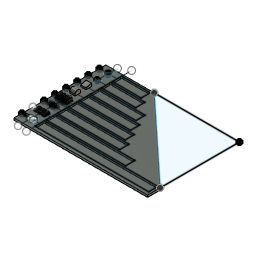
tactileMapsLegend (Autodesk Fusion 360 archive; units mm, degrees)
design "tactileMapsLegendApril26" references "TactileMapsParameters"
Autodesk Fusion 360 part; units mm, degrees
derive "ExternalDerived1" from "TactileMapsParameters v7"
sketch "Sketch1" plane through (0, 0, 0) normal (0, 0, 1) x (1, 0, 0)
  line L0 (0, 0) -> (147.25, 0)
  line L1 (147.25, 0) -> (147.25, 101.2)
  line L2 (147.25, 101.2) -> (0, 101.2)
  line L3 (0, 101.2) -> (0, 0)
  dimension "d21" = 147.25
  dimension "d22" = 101.2
  constraint horizontal L0
  constraint vertical L1
  constraint horizontal L2
  constraint vertical L3
  constraint coincident L0.start L3.end
  measures "d21" distance of L0.start L0.end
  measures "d22" distance of L0.start L2.end
extrude "Extrude1" add sketch "Sketch1" along normal blind 2.2
sketch "Sketch2" plane through (0, 0, 2.2) normal (0, 0, 1) x (-1, 0, 0)
  line L0 (0, -101.2) -> (0, 0)
  line L1 (0, 0) -> (-147.25, 0)
  line L2 (-147.25, 0) -> (-147.25, -101.2)
  line L3 (-147.25, -101.2) -> (0, -101.2)
  line L4 (-19.6, -110.066) -> (-19.6, 6.0036) construction
  line L5 (-19.6, -99.2) -> (-51.05, -99.2)
  line L6 (-51.05, -99.2) -> (-51.05, -89)
  line L7 (-51.05, -89) -> (-19.6, -89)
  line L8 (-19.6, -89) -> (-19.6, -99.2)
  line L9 (-19.6, -87) -> (-57.3, -87)
  line L10 (-57.3, -87) -> (-57.3, -76.8)
  line L11 (-57.3, -76.8) -> (-19.6, -76.8)
  line L12 (-19.6, -76.8) -> (-19.6, -87)
  line L13 (-19.6, -74.8) -> (-69.8, -74.8)
  line L14 (-69.8, -74.8) -> (-69.8, -64.6)
  line L15 (-69.8, -64.6) -> (-19.6, -64.6)
  line L16 (-19.6, -64.6) -> (-19.6, -74.8)
  line L17 (-19.6, -62.6) -> (-76.05, -62.6)
  line L18 (-76.05, -62.6) -> (-76.05, -52.4)
  line L19 (-76.05, -52.4) -> (-19.6, -52.4)
  line L20 (-19.6, -52.4) -> (-19.6, -62.6)
  line L21 (-19.6, -50.4) -> (-82.3, -50.4)
  line L22 (-82.3, -50.4) -> (-82.3, -40.2)
  line L23 (-82.3, -40.2) -> (-19.6, -40.2)
  line L24 (-19.6, -40.2) -> (-19.6, -50.4)
  line L25 (-19.6, -38.2) -> (-88.55, -38.2)
  line L26 (-88.55, -38.2) -> (-88.55, -28)
  line L27 (-88.55, -28) -> (-19.6, -28)
  line L28 (-19.6, -28) -> (-19.6, -38.2)
  line L29 (-19.6, -26) -> (-107.3, -26)
  line L30 (-107.3, -26) -> (-107.3, -15.8)
  line L31 (-107.3, -15.8) -> (-19.6, -15.8)
  line L32 (-19.6, -15.8) -> (-19.6, -26)
  line L33 (-19.6, -13.8) -> (-144.8, -13.8)
  line L34 (-144.8, -13.8) -> (-144.8, -3.6)
  line L35 (-144.8, -3.6) -> (-19.6, -3.6)
  line L36 (-19.6, -3.6) -> (-19.6, -13.8)
  line L37 (-19.6, -94.1) -> (0, -94.1) construction
  line L38 (-19.6, -81.9) -> (0, -81.9) construction
  line L39 (-19.6, -69.7) -> (0, -69.7) construction
  line L40 (-19.6, -57.5) -> (0, -57.5) construction
  line L41 (-19.6, -45.3) -> (0, -45.3) construction
  line L42 (-19.6, -33.1) -> (0, -33.1) construction
  line L43 (-19.6, -20.9) -> (0, -20.9) construction
  line L44 (-19.6, -8.7) -> (0, -8.7) construction
  line L45 (-11.8835, -96.2585) -> (-9.747, -97.0995)
  line L46 (-9.747, -97.0995) -> (-7.6415, -96.1835)
  line L47 (-7.6415, -96.1835) -> (-6.8005, -94.047)
  line L48 (-6.8005, -94.047) -> (-7.7165, -91.9415)
  line L49 (-7.7165, -91.9415) -> (-9.853, -91.1005)
  line L50 (-9.853, -91.1005) -> (-11.9585, -92.0165)
  line L51 (-11.9585, -92.0165) -> (-12.7995, -94.153)
  line L52 (-12.7995, -94.153) -> (-11.8835, -96.2585)
  line L53 (-12.3958, -83.4039) -> (-7.1997, -83.3961)
  line L54 (-7.1997, -83.3961) -> (-9.8045, -78.9)
  line L55 (-9.8045, -78.9) -> (-12.3958, -83.4039)
  line L56 (-15.8, -48.3) -> (-3.8, -48.3)
  line L57 (-3.8, -48.3) -> (-3.8, -42.3)
  line L58 (-3.8, -42.3) -> (-15.8, -42.3)
  line L59 (-15.8, -42.3) -> (-15.8, -48.3)
  line L60 (-15.8, -48.3) -> (-3.8, -42.3) construction
  line L61 (-3.8, -48.3) -> (-15.8, -42.3) construction
  line L62 (-3.8, -48.3) -> (-5.3, -48.3)
  line L63 (-5.3, -48.3) -> (-5.3, -42.3)
  line L64 (-5.3, -42.3) -> (-3.8, -42.3)
  line L65 (-3.8, -42.3) -> (-3.8, -48.3)
  line L66 (-8.8, -48.3) -> (-8.8, -42.3)
  line L67 (-7.3, -48.3) -> (-7.3, -42.3)
  line L68 (-7.3, -48.3) -> (-8.8, -48.3)
  line L69 (-8.8, -42.3) -> (-7.3, -42.3)
  line L70 (-12.3, -48.3) -> (-12.3, -42.3)
  line L71 (-10.8, -48.3) -> (-10.8, -42.3)
  line L72 (-10.8, -48.3) -> (-12.3, -48.3)
  line L73 (-12.3, -42.3) -> (-10.8, -42.3)
  line L74 (-15.8, -48.3) -> (-15.8, -42.3)
  line L75 (-14.3, -48.3) -> (-14.3, -42.3)
  line L76 (-14.3, -48.3) -> (-15.8, -48.3)
  line L77 (-15.8, -42.3) -> (-14.3, -42.3)
  circle A0 centre (-9.8, -33.1) radius 0.75
  circle A1 centre (-12.8, -33.1) radius 0.75
  circle A2 centre (-6.8, -33.1) radius 0.75
  line L78 (-3.8, -23.4) -> (-15.8, -23.4)
  line L79 (-15.8, -23.4) -> (-15.8, -21.9)
  line L80 (-15.8, -21.9) -> (-3.8, -21.9)
  line L81 (-3.8, -21.9) -> (-3.8, -23.4)
  line L82 (-15.8, -19.9) -> (-3.8, -19.9)
  line L83 (-3.8, -19.9) -> (-3.8, -18.4)
  line L84 (-3.8, -18.4) -> (-15.8, -18.4)
  line L85 (-15.8, -18.4) -> (-15.8, -19.9)
  line L86 (-4.8, -23.9) -> (-6.3, -23.9)
  line L87 (-6.3, -23.9) -> (-6.3, -17.9)
  line L88 (-6.3, -17.9) -> (-4.8, -17.9)
  line L89 (-4.8, -17.9) -> (-4.8, -23.9)
  line L90 (-10.55, -23.9) -> (-10.55, -17.9)
  line L91 (-9.05, -23.9) -> (-10.55, -23.9)
  line L92 (-9.05, -17.9) -> (-9.05, -23.9)
  line L93 (-10.55, -17.9) -> (-9.05, -17.9)
  line L94 (-14.8, -23.9) -> (-14.8, -17.9)
  line L95 (-13.3, -23.9) -> (-14.8, -23.9)
  line L96 (-13.3, -17.9) -> (-13.3, -23.9)
  line L97 (-14.8, -17.9) -> (-13.3, -17.9)
  line L98 (-3.8, -9.7) -> (-9.9716, -9.7)
  line L99 (-9.9716, -7.7) -> (-3.8, -7.7)
  line L100 (-3.8, -7.7) -> (-3.8, -9.7)
  arc A3 (-9.9716, -7.7) -> (-9.9716, -9.7) centre (-12.8, -8.7) ccw
  line L101 (-9.8, -104.251) -> (-9.8, -8.7) construction
  line L102 (-9.8, -7.7) -> (-9.8, 5.278) construction
  line L103 (-53.2749, -101.2) -> (-147.25, -13.8)
  line L104 (-147.25, -13.8) -> (-147.25, -101.2)
  line L105 (-147.25, -101.2) -> (-53.2749, -101.2)
  point P0 (-9.8, -94.1)
  point P1 (-9.8, -81.9)
  point P2 (-9.8, -45.3)
  dimension "d25" = 19.6
  dimension "d26" = 31.45
  dimension "d27" = 10.2
  dimension "d28" = 2
  dimension "d29" = 37.7
  dimension "d30" = 2
  dimension "d31" = 10.2
  dimension "d32" = 50.2
  dimension "d33" = 10.2
  dimension "d34" = 2
  dimension "d35" = 56.45
  dimension "d36" = 10.2
  dimension "d37" = 2
  dimension "d38" = 62.7
  dimension "d39" = 10.2
  dimension "d40" = 2
  dimension "d41" = 68.95
  dimension "d42" = 10.2
  dimension "d43" = 2
  dimension "d44" = 87.7
  dimension "d45" = 10.2
  dimension "d46" = 2
  dimension "d47" = 125.2
  dimension "d48" = 10.2
  dimension "d49" = 2
  dimension "d50" = 9.8
  dimension "d51" = 3
  dimension "d52" = 3
  dimension "d53" = 12
  dimension "d54" = 6
  dimension "d55" = 1.5
  dimension "d56" = 6
  dimension "d59" = -10.5
  dimension "d60" = 0
  dimension "d61" = 1.5
  dimension "d64" = 3
  dimension "d65" = 0
  dimension "d66" = 12
  dimension "d67" = 1.5
  dimension "d68" = 6
  dimension "d69" = 2.5
  dimension "d70" = 1.5
  dimension "d71" = 6
  dimension "d72" = 0.5
  dimension "d73" = 1
  dimension "d76" = -8.5
  dimension "d77" = 0
  dimension "d78" = 6
  dimension "d83" = 2
  dimension "d84" = 1
  dimension "d85" = 6
  constraint perpendicular L1 L4
  constraint horizontal L5
  constraint vertical L6
  constraint horizontal L7
  constraint vertical L8
  constraint coincident L4 L5.start
  constraint horizontal L9
  constraint vertical L10
  constraint horizontal L11
  constraint vertical L12
  constraint coincident L4 L9.start
  constraint horizontal L13
  constraint vertical L14
  constraint horizontal L15
  constraint vertical L16
  constraint coincident L4 L13.start
  constraint horizontal L17
  constraint vertical L18
  constraint horizontal L19
  constraint vertical L20
  constraint coincident L4 L17.start
  constraint horizontal L21
  constraint vertical L22
  constraint horizontal L23
  constraint vertical L24
  constraint coincident L4 L21.start
  constraint horizontal L25
  constraint vertical L26
  constraint horizontal L27
  constraint vertical L28
  constraint coincident L4 L25.start
  constraint horizontal L29
  constraint vertical L30
  constraint horizontal L31
  constraint vertical L32
  constraint coincident L4 L29.start
  constraint horizontal L33
  constraint vertical L34
  constraint horizontal L35
  constraint vertical L36
  constraint coincident L4 L33.start
  constraint perpendicular L1 L101
  constraint midpoint L8 L37.start
  constraint coincident L0 L37.end
  constraint perpendicular L0 L37
  constraint midpoint L12 L38.start
  constraint coincident L0 L38.end
  constraint perpendicular L0 L38
  constraint midpoint L16 L39.start
  constraint coincident L0 L39.end
  constraint perpendicular L0 L39
  constraint midpoint L20 L40.start
  constraint coincident L0 L40.end
  constraint perpendicular L0 L40
  constraint midpoint L24 L41.start
  constraint coincident L0 L41.end
  constraint perpendicular L0 L41
  constraint midpoint L28 L42.start
  constraint coincident L0 L42.end
  constraint perpendicular L0 L42
  constraint midpoint L32 L43.start
  constraint perpendicular L32 L43
  constraint midpoint L36 L44.start
  constraint coincident L0 L44.end
  constraint perpendicular L0 L44
  constraint midpoint L37 P0
  constraint midpoint L38 P1
  constraint horizontal L56
  constraint perpendicular L56 L57
  constraint parallel L56 L58
  constraint parallel L57 L59
  constraint coincident L60 P2
  constraint coincident L61 P2
  constraint midpoint L41 P2
  constraint horizontal L62
  constraint vertical L63
  constraint horizontal L64
  constraint vertical L65
  constraint midpoint L42 A0.centre
  constraint horizontal L78
  constraint vertical L79
  constraint horizontal L80
  constraint vertical L81
  constraint symmetric L43 L78.start L83.end
  constraint symmetric L43 L78.end L84.end
  constraint symmetric L43 L79.end L82.start
  constraint symmetric L43 L80.end L82.end
  constraint horizontal L86
  constraint vertical L87
  constraint horizontal L88
  constraint vertical L89
  constraint horizontal L98
  constraint horizontal L99
  constraint vertical L100
  constraint coincident L102.start L99
  constraint collinear L101 L102
  constraint coincident L3 L103.start
  constraint coincident L2 L103.end
  constraint coincident L2.end L3.start
  measures "d25" distance of L0 L4
  measures "d26" distance of L5.start L5.end
  measures "d27" distance of L5.start L7.end
  measures "d28" distance of L3 L5
  measures "d29" distance of L9.start L9.end
  measures "d30" distance of L7 L9
  measures "d31" distance of L9.end L10.end
  measures "d32" distance of L13.start L13.end
  measures "d33" distance of L13.start L15.end
  measures "d34" distance of L11 L13
  measures "d35" distance of L17.start L17.end
  measures "d36" distance of L17.start L19.end
  measures "d37" distance of L15 L17
  measures "d38" distance of L21.start L21.end
  measures "d39" distance of L21.start L23.end
  measures "d40" distance of L19 L21
  measures "d41" distance of L25.start L25.end
  measures "d42" distance of L25.start L27.end
  measures "d43" distance of L23 L25
  measures "d44" distance of L29.start L29.end
  measures "d45" distance of L29.start L31.end
  measures "d46" distance of L27 L29
  measures "d47" distance of L33.start L33.end
  measures "d48" distance of L33.start L35.end
  measures "d49" distance of L31 L33
  measures "d50" distance of L0.start L101
  measures "d51" distance of L45.start P0
  measures "d52" distance of L53.start P1
  measures "d53" distance of L57.end L58.end
  measures "d54" distance of L56.end L57.end
  measures "d55" distance of L56.end L62.end
  measures "d56" distance of L56.end L57.end
  measures "d61" diameter of A0
  measures "d66" distance of L78.start L78.end
  measures "d67" distance of L78.start L80.end
  measures "d68" distance of L81 L101
  measures "d69" distance of L43 L78
  measures "d70" distance of L86.start L86.end
  measures "d71" distance of L86.start L88.end
  measures "d72" distance of L78 L86
  measures "d73" distance of L83 L89
  measures "d78" diameter of A3
  measures "d83" distance of L98.start L99.end
  measures "d84" distance of L44 L98
  measures "d85" distance of L100 L101
extrude "Extrude2" cut sketch "Sketch2" against normal blind 2 contours L5 L6 L7 L8 | L9 L10 L11 L12 | L13 L14 L15 L16 | L17 L18 L19 L20 | L21 L22 L23 L24 | L25 L26 L27 L28 | L29 L30 L31 L32 | L33 L34 L35 L36
ref_plane "WorkPlane1" through (88.55, 38.2, 2.2) normal (0, 0, -1) x (-1, 0, 0)
sketch "Sketch3" plane through (88.55, 38.2, 2.2) normal (0, 0, -1) x (-1, 0, 0)
  line L0 (68.95, 0) -> (0, 0) construction
  line L1 (0, 0) -> (0, -10.2) construction
  line L2 (0, 0) -> (0.7071, -0.7071) construction
  circle A0 centre (0.7071, -0.7071) radius 1
  dimension "d89" = 1
  constraint coincident L0.end L1.start
  constraint coincident L0.end A0
  measures "d89" distance of L0.end L2.end
sweep "Sweep1" cut kept parallel profiles "Sketch3" along 1 edges at (88.55, 38.2, 1.2) section 1
ref_plane "WorkPlane2" through (88.55, 28, 2.2) normal (0, 0, -1) x (-1, 0, 0)
sketch "Sketch4" plane through (88.55, 28, 2.2) normal (0, 0, -1) x (-1, 0, 0)
  line L0 (0, 0) -> (68.95, 0) construction
  line L1 (0, 8.7858) -> (0, 0) construction
  line L2 (0, 0) -> (0.7071, 0.7071) construction
  circle A0 centre (0.7071, 0.7071) radius 1
  dimension "d97" = 1
  constraint coincident L0.start L1.end
  constraint coincident L0.start A0
  measures "d97" distance of L0.start L2.end
sweep "Sweep2" cut kept parallel profiles "Sketch4" along 1 edges at (88.55, 28, 1.2) section 1
ref_plane "WorkPlane3" through (19.6, 38.2, 2.2) normal (0, 0, -1) x (-1, 0, 0)
sketch "Sketch5" plane through (19.6, 38.2, 2.2) normal (0, 0, -1) x (-1, 0, 0)
  line L0 (0, -10.2) -> (0, 0) construction
  line L1 (0, 0) -> (-67.5358, 0) construction
  line L2 (0, 0) -> (-0.7071, -0.7071) construction
  circle A0 centre (-0.7071, -0.7071) radius 1
  dimension "d105" = 1
  constraint coincident L0.end L1.start
  constraint coincident L0.end A0
  measures "d105" distance of L0.end L2.end
sweep "Sweep3" cut kept parallel profiles "Sketch5" along 1 edges at (19.6, 38.2, 1.2) section 1
ref_plane "WorkPlane4" through (19.6, 28, 2.2) normal (0, 0, -1) x (-1, 0, 0)
sketch "Sketch6" plane through (19.6, 28, 2.2) normal (0, 0, -1) x (-1, 0, 0)
  line L0 (-67.5358, 0) -> (0, 0) construction
  line L1 (0, 0) -> (0, 8.7858) construction
  line L2 (0, 0) -> (-0.7071, 0.7071) construction
  circle A0 centre (-0.7071, 0.7071) radius 1
  dimension "d113" = 1
  constraint coincident L0.end L1.start
  constraint coincident L0.end A0
  measures "d113" distance of L0.end L2.end
sweep "Sweep4" cut kept parallel profiles "Sketch6" along 1 edges at (19.6, 28, 1.2) section 1
ref_plane "WorkPlane5" through (57.3, 87, 2.2) normal (0, 0, -1) x (-1, 0, 0)
sketch "Sketch7" plane through (57.3, 87, 2.2) normal (0, 0, -1) x (-1, 0, 0)
  line L0 (37.7, 0) -> (0, 0) construction
  line L1 (0, 0) -> (0, -10.2) construction
  line L2 (0, 0) -> (0.7071, -0.7071) construction
  circle A0 centre (0.7071, -0.7071) radius 1
  dimension "d121" = 1
  constraint coincident L0.end L1.start
  constraint coincident L0.end A0
  measures "d121" distance of L0.end L2.end
sweep "Sweep5" cut kept parallel profiles "Sketch7" along 1 edges at (57.3, 87, 1.2) section 1
ref_plane "WorkPlane6" through (57.3, 76.8, 2.2) normal (0, 0, -1) x (-1, 0, 0)
sketch "Sketch8" plane through (57.3, 76.8, 2.2) normal (0, 0, -1) x (-1, 0, 0)
  line L0 (0, 0) -> (37.7, 0) construction
  line L1 (0, 8.7858) -> (0, 0) construction
  line L2 (0, 0) -> (0.7071, 0.7071) construction
  circle A0 centre (0.7071, 0.7071) radius 1
  dimension "d129" = 1
  constraint coincident L0.start L1.end
  constraint coincident L0.start A0
  measures "d129" distance of L0.start L2.end
sweep "Sweep6" cut kept parallel profiles "Sketch8" along 1 edges at (57.3, 76.8, 1.2) section 1
ref_plane "WorkPlane7" through (19.6, 87, 2.2) normal (0, 0, -1) x (-1, 0, 0)
sketch "Sketch9" plane through (19.6, 87, 2.2) normal (0, 0, -1) x (-1, 0, 0)
  line L0 (0, -10.2) -> (0, 0) construction
  line L1 (0, 0) -> (-36.2858, 0) construction
  line L2 (0, 0) -> (-0.7071, -0.7071) construction
  circle A0 centre (-0.7071, -0.7071) radius 1
  dimension "d137" = 1
  constraint coincident L0.end L1.start
  constraint coincident L0.end A0
  measures "d137" distance of L0.end L2.end
sweep "Sweep7" cut kept parallel profiles "Sketch9" along 1 edges at (19.6, 87, 1.2) section 1
ref_plane "WorkPlane8" through (19.6, 76.8, 2.2) normal (0, 0, -1) x (-1, 0, 0)
sketch "Sketch10" plane through (19.6, 76.8, 2.2) normal (0, 0, -1) x (-1, 0, 0)
  line L0 (-36.2858, 0) -> (0, 0) construction
  line L1 (0, 0) -> (0, 8.7858) construction
  line L2 (0, 0) -> (-0.7071, 0.7071) construction
  circle A0 centre (-0.7071, 0.7071) radius 1
  dimension "d145" = 1
  constraint coincident L0.end L1.start
  constraint coincident L0.end A0
  measures "d145" distance of L0.end L2.end
sweep "Sweep8" cut kept parallel profiles "Sketch10" along 1 edges at (19.6, 76.8, 1.2) section 1
ref_plane "WorkPlane9" through (69.8, 74.8, 2.2) normal (0, 0, -1) x (-1, 0, 0)
sketch "Sketch11" plane through (69.8, 74.8, 2.2) normal (0, 0, -1) x (-1, 0, 0)
  line L0 (50.2, 0) -> (0, 0) construction
  line L1 (0, 0) -> (0, -10.2) construction
  line L2 (0, 0) -> (0.7071, -0.7071) construction
  circle A0 centre (0.7071, -0.7071) radius 1
  dimension "d153" = 1
  constraint coincident L0.end L1.start
  constraint coincident L0.end A0
  measures "d153" distance of L0.end L2.end
sweep "Sweep9" cut kept parallel profiles "Sketch11" along 1 edges at (69.8, 74.8, 1.2) section 1
ref_plane "WorkPlane10" through (69.8, 64.6, 2.2) normal (0, 0, -1) x (-1, 0, 0)
sketch "Sketch12" plane through (69.8, 64.6, 2.2) normal (0, 0, -1) x (-1, 0, 0)
  line L0 (0, 0) -> (50.2, 0) construction
  line L1 (0, 8.7858) -> (0, 0) construction
  line L2 (0, 0) -> (0.7071, 0.7071) construction
  circle A0 centre (0.7071, 0.7071) radius 1
  dimension "d161" = 1
  constraint coincident L0.start L1.end
  constraint coincident L0.start A0
  measures "d161" distance of L0.start L2.end
sweep "Sweep10" cut kept parallel profiles "Sketch12" along 1 edges at (69.8, 64.6, 1.2) section 1
ref_plane "WorkPlane11" through (19.6, 74.8, 2.2) normal (0, 0, -1) x (-1, 0, 0)
sketch "Sketch13" plane through (19.6, 74.8, 2.2) normal (0, 0, -1) x (-1, 0, 0)
  line L0 (0, -10.2) -> (0, 0) construction
  line L1 (0, 0) -> (-48.7858, 0) construction
  line L2 (0, 0) -> (-0.7071, -0.7071) construction
  circle A0 centre (-0.7071, -0.7071) radius 1
  dimension "d169" = 1
  constraint coincident L0.end L1.start
  constraint coincident L0.end A0
  measures "d169" distance of L0.end L2.end
sweep "Sweep11" cut kept parallel profiles "Sketch13" along 1 edges at (19.6, 74.8, 1.2) section 1
ref_plane "WorkPlane12" through (19.6, 64.6, 2.2) normal (0, 0, -1) x (-1, 0, 0)
sketch "Sketch14" plane through (19.6, 64.6, 2.2) normal (0, 0, -1) x (-1, 0, 0)
  line L0 (-48.7858, 0) -> (0, 0) construction
  line L1 (0, 0) -> (0, 8.7858) construction
  line L2 (0, 0) -> (-0.7071, 0.7071) construction
  circle A0 centre (-0.7071, 0.7071) radius 1
  dimension "d177" = 1
  constraint coincident L0.end L1.start
  constraint coincident L0.end A0
  measures "d177" distance of L0.end L2.end
sweep "Sweep12" cut kept parallel profiles "Sketch14" along 1 edges at (19.6, 64.6, 1.2) section 1
ref_plane "WorkPlane13" through (107.3, 26, 2.2) normal (0, 0, -1) x (-1, 0, 0)
sketch "Sketch15" plane through (107.3, 26, 2.2) normal (0, 0, -1) x (-1, 0, 0)
  line L0 (87.7, 0) -> (0, 0) construction
  line L1 (0, 0) -> (0, -10.2) construction
  line L2 (0, 0) -> (0.7071, -0.7071) construction
  circle A0 centre (0.7071, -0.7071) radius 1
  dimension "d185" = 1
  constraint coincident L0.end L1.start
  constraint coincident L0.end A0
  measures "d185" distance of L0.end L2.end
sweep "Sweep13" cut kept parallel profiles "Sketch15" along 1 edges at (107.3, 26, 1.2) section 1
ref_plane "WorkPlane14" through (107.3, 15.8, 2.2) normal (0, 0, -1) x (-1, 0, 0)
sketch "Sketch16" plane through (107.3, 15.8, 2.2) normal (0, 0, -1) x (-1, 0, 0)
  line L0 (0, 0) -> (87.7, 0) construction
  line L1 (0, 8.7858) -> (0, 0) construction
  line L2 (0, 0) -> (0.7071, 0.7071) construction
  circle A0 centre (0.7071, 0.7071) radius 1
  dimension "d193" = 1
  constraint coincident L0.start L1.end
  constraint coincident L0.start A0
  measures "d193" distance of L0.start L2.end
sweep "Sweep14" cut kept parallel profiles "Sketch16" along 1 edges at (107.3, 15.8, 1.2) section 1
ref_plane "WorkPlane15" through (19.6, 26, 2.2) normal (0, 0, -1) x (-1, 0, 0)
sketch "Sketch17" plane through (19.6, 26, 2.2) normal (0, 0, -1) x (-1, 0, 0)
  line L0 (0, -10.2) -> (0, 0) construction
  line L1 (0, 0) -> (-86.2858, 0) construction
  line L2 (0, 0) -> (-0.7071, -0.7071) construction
  circle A0 centre (-0.7071, -0.7071) radius 1
  dimension "d201" = 1
  constraint coincident L0.end L1.start
  constraint coincident L0.end A0
  measures "d201" distance of L0.end L2.end
sweep "Sweep15" cut kept parallel profiles "Sketch17" along 1 edges at (19.6, 26, 1.2) section 1
ref_plane "WorkPlane16" through (19.6, 15.8, 2.2) normal (0, 0, -1) x (-1, 0, 0)
sketch "Sketch18" plane through (19.6, 15.8, 2.2) normal (0, 0, -1) x (-1, 0, 0)
  line L0 (-86.2858, 0) -> (0, 0) construction
  line L1 (0, 0) -> (0, 8.7858) construction
  line L2 (0, 0) -> (-0.7071, 0.7071) construction
  circle A0 centre (-0.7071, 0.7071) radius 1
  dimension "d209" = 1
  constraint coincident L0.end L1.start
  constraint coincident L0.end A0
  measures "d209" distance of L0.end L2.end
sweep "Sweep16" cut kept parallel profiles "Sketch18" along 1 edges at (19.6, 15.8, 1.2) section 1
ref_plane "WorkPlane17" through (82.3, 50.4, 2.2) normal (0, 0, -1) x (-1, 0, 0)
sketch "Sketch19" plane through (82.3, 50.4, 2.2) normal (0, 0, -1) x (-1, 0, 0)
  line L0 (62.7, 0) -> (0, 0) construction
  line L1 (0, 0) -> (0, -10.2) construction
  line L2 (0, 0) -> (0.7071, -0.7071) construction
  circle A0 centre (0.7071, -0.7071) radius 1
  dimension "d217" = 1
  constraint coincident L0.end L1.start
  constraint coincident L0.end A0
  measures "d217" distance of L0.end L2.end
sweep "Sweep17" cut kept parallel profiles "Sketch19" along 1 edges at (82.3, 50.4, 1.2) section 1
ref_plane "WorkPlane18" through (82.3, 40.2, 2.2) normal (0, 0, -1) x (-1, 0, 0)
sketch "Sketch20" plane through (82.3, 40.2, 2.2) normal (0, 0, -1) x (-1, 0, 0)
  line L0 (0, 0) -> (62.7, 0) construction
  line L1 (0, 8.7858) -> (0, 0) construction
  line L2 (0, 0) -> (0.7071, 0.7071) construction
  circle A0 centre (0.7071, 0.7071) radius 1
  dimension "d225" = 1
  constraint coincident L0.start L1.end
  constraint coincident L0.start A0
  measures "d225" distance of L0.start L2.end
sweep "Sweep18" cut kept parallel profiles "Sketch20" along 1 edges at (82.3, 40.2, 1.2) section 1
ref_plane "WorkPlane19" through (19.6, 50.4, 2.2) normal (0, 0, -1) x (-1, 0, 0)
sketch "Sketch21" plane through (19.6, 50.4, 2.2) normal (0, 0, -1) x (-1, 0, 0)
  line L0 (0, -10.2) -> (0, 0) construction
  line L1 (0, 0) -> (-61.2858, 0) construction
  line L2 (0, 0) -> (-0.7071, -0.7071) construction
  circle A0 centre (-0.7071, -0.7071) radius 1
  dimension "d233" = 1
  constraint coincident L0.end L1.start
  constraint coincident L0.end A0
  measures "d233" distance of L0.end L2.end
sweep "Sweep19" cut kept parallel profiles "Sketch21" along 1 edges at (19.6, 50.4, 1.2) section 1
ref_plane "WorkPlane20" through (19.6, 40.2, 2.2) normal (0, 0, -1) x (-1, 0, 0)
sketch "Sketch22" plane through (19.6, 40.2, 2.2) normal (0, 0, -1) x (-1, 0, 0)
  line L0 (-61.2858, 0) -> (0, 0) construction
  line L1 (0, 0) -> (0, 8.7858) construction
  line L2 (0, 0) -> (-0.7071, 0.7071) construction
  circle A0 centre (-0.7071, 0.7071) radius 1
  dimension "d241" = 1
  constraint coincident L0.end L1.start
  constraint coincident L0.end A0
  measures "d241" distance of L0.end L2.end
sweep "Sweep20" cut kept parallel profiles "Sketch22" along 1 edges at (19.6, 40.2, 1.2) section 1
ref_plane "WorkPlane21" through (51.05, 99.2, 2.2) normal (0, 0, -1) x (-1, 0, 0)
sketch "Sketch23" plane through (51.05, 99.2, 2.2) normal (0, 0, -1) x (-1, 0, 0)
  line L0 (31.45, 0) -> (0, 0) construction
  line L1 (0, 0) -> (0, -10.2) construction
  line L2 (0, 0) -> (0.7071, -0.7071) construction
  circle A0 centre (0.7071, -0.7071) radius 1
  dimension "d249" = 1
  constraint coincident L0.end L1.start
  constraint coincident L0.end A0
  measures "d249" distance of L0.end L2.end
sweep "Sweep21" cut kept parallel profiles "Sketch23" along 1 edges at (51.05, 99.2, 1.2) section 1
ref_plane "WorkPlane22" through (51.05, 89, 2.2) normal (0, 0, -1) x (-1, 0, 0)
sketch "Sketch24" plane through (51.05, 89, 2.2) normal (0, 0, -1) x (-1, 0, 0)
  line L0 (0, 0) -> (31.45, 0) construction
  line L1 (0, 8.7858) -> (0, 0) construction
  line L2 (0, 0) -> (0.7071, 0.7071) construction
  circle A0 centre (0.7071, 0.7071) radius 1
  dimension "d257" = 1
  constraint coincident L0.start L1.end
  constraint coincident L0.start A0
  measures "d257" distance of L0.start L2.end
sweep "Sweep22" cut kept parallel profiles "Sketch24" along 1 edges at (51.05, 89, 1.2) section 1
ref_plane "WorkPlane23" through (19.6, 99.2, 2.2) normal (0, 0, -1) x (-1, 0, 0)
sketch "Sketch25" plane through (19.6, 99.2, 2.2) normal (0, 0, -1) x (-1, 0, 0)
  line L0 (0, -10.2) -> (0, 0) construction
  line L1 (0, 0) -> (-30.0358, 0) construction
  line L2 (0, 0) -> (-0.7071, -0.7071) construction
  circle A0 centre (-0.7071, -0.7071) radius 1
  dimension "d265" = 1
  constraint coincident L0.end L1.start
  constraint coincident L0.end A0
  measures "d265" distance of L0.end L2.end
sweep "Sweep23" cut kept parallel profiles "Sketch25" along 1 edges at (19.6, 99.2, 1.2) section 1
ref_plane "WorkPlane24" through (19.6, 89, 2.2) normal (0, 0, -1) x (-1, 0, 0)
sketch "Sketch26" plane through (19.6, 89, 2.2) normal (0, 0, -1) x (-1, 0, 0)
  line L0 (-30.0358, 0) -> (0, 0) construction
  line L1 (0, 0) -> (0, 8.7858) construction
  line L2 (0, 0) -> (-0.7071, 0.7071) construction
  circle A0 centre (-0.7071, 0.7071) radius 1
  dimension "d273" = 1
  constraint coincident L0.end L1.start
  constraint coincident L0.end A0
  measures "d273" distance of L0.end L2.end
sweep "Sweep24" cut kept parallel profiles "Sketch26" along 1 edges at (19.6, 89, 1.2) section 1
ref_plane "WorkPlane25" through (76.05, 62.6, 2.2) normal (0, 0, -1) x (-1, 0, 0)
sketch "Sketch27" plane through (76.05, 62.6, 2.2) normal (0, 0, -1) x (-1, 0, 0)
  line L0 (56.45, 0) -> (0, 0) construction
  line L1 (0, 0) -> (0, -10.2) construction
  line L2 (0, 0) -> (0.7071, -0.7071) construction
  circle A0 centre (0.7071, -0.7071) radius 1
  dimension "d281" = 1
  constraint coincident L0.end L1.start
  constraint coincident L0.end A0
  measures "d281" distance of L0.end L2.end
sweep "Sweep25" cut kept parallel profiles "Sketch27" along 1 edges at (76.05, 62.6, 1.2) section 1
ref_plane "WorkPlane26" through (76.05, 52.4, 2.2) normal (0, 0, -1) x (-1, 0, 0)
sketch "Sketch28" plane through (76.05, 52.4, 2.2) normal (0, 0, -1) x (-1, 0, 0)
  line L0 (0, 0) -> (56.45, 0) construction
  line L1 (0, 8.7858) -> (0, 0) construction
  line L2 (0, 0) -> (0.7071, 0.7071) construction
  circle A0 centre (0.7071, 0.7071) radius 1
  dimension "d289" = 1
  constraint coincident L0.start L1.end
  constraint coincident L0.start A0
  measures "d289" distance of L0.start L2.end
sweep "Sweep26" cut kept parallel profiles "Sketch28" along 1 edges at (76.05, 52.4, 1.2) section 1
ref_plane "WorkPlane27" through (19.6, 62.6, 2.2) normal (0, 0, -1) x (-1, 0, 0)
sketch "Sketch29" plane through (19.6, 62.6, 2.2) normal (0, 0, -1) x (-1, 0, 0)
  line L0 (0, -10.2) -> (0, 0) construction
  line L1 (0, 0) -> (-55.0358, 0) construction
  line L2 (0, 0) -> (-0.7071, -0.7071) construction
  circle A0 centre (-0.7071, -0.7071) radius 1
  dimension "d297" = 1
  constraint coincident L0.end L1.start
  constraint coincident L0.end A0
  measures "d297" distance of L0.end L2.end
sweep "Sweep27" cut kept parallel profiles "Sketch29" along 1 edges at (19.6, 62.6, 1.2) section 1
ref_plane "WorkPlane28" through (19.6, 52.4, 2.2) normal (0, 0, -1) x (-1, 0, 0)
sketch "Sketch30" plane through (19.6, 52.4, 2.2) normal (0, 0, -1) x (-1, 0, 0)
  line L0 (-55.0358, 0) -> (0, 0) construction
  line L1 (0, 0) -> (0, 8.7858) construction
  line L2 (0, 0) -> (-0.7071, 0.7071) construction
  circle A0 centre (-0.7071, 0.7071) radius 1
  dimension "d305" = 1
  constraint coincident L0.end L1.start
  constraint coincident L0.end A0
  measures "d305" distance of L0.end L2.end
sweep "Sweep28" cut kept parallel profiles "Sketch30" along 1 edges at (19.6, 52.4, 1.2) section 1
ref_plane "WorkPlane29" through (144.8, 13.8, 2.2) normal (0, 0, -1) x (-1, 0, 0)
sketch "Sketch31" plane through (144.8, 13.8, 2.2) normal (0, 0, -1) x (-1, 0, 0)
  line L0 (125.2, 0) -> (0, 0) construction
  line L1 (0, 0) -> (0, -10.2) construction
  line L2 (0, 0) -> (0.7071, -0.7071) construction
  circle A0 centre (0.7071, -0.7071) radius 1
  dimension "d313" = 1
  constraint coincident L0.end L1.start
  constraint coincident L0.end A0
  measures "d313" distance of L0.end L2.end
sweep "Sweep29" cut kept parallel profiles "Sketch31" along 1 edges at (144.8, 13.8, 1.2) section 1
ref_plane "WorkPlane30" through (144.8, 3.6, 2.2) normal (0, 0, -1) x (-1, 0, 0)
sketch "Sketch32" plane through (144.8, 3.6, 2.2) normal (0, 0, -1) x (-1, 0, 0)
  line L0 (0, 0) -> (125.2, 0) construction
  line L1 (0, 8.7858) -> (0, 0) construction
  line L2 (0, 0) -> (0.7071, 0.7071) construction
  circle A0 centre (0.7071, 0.7071) radius 1
  dimension "d321" = 1
  constraint coincident L0.start L1.end
  constraint coincident L0.start A0
  measures "d321" distance of L0.start L2.end
sweep "Sweep30" cut kept parallel profiles "Sketch32" along 1 edges at (144.8, 3.6, 1.2) section 1
ref_plane "WorkPlane31" through (19.6, 13.8, 2.2) normal (0, 0, -1) x (-1, 0, 0)
sketch "Sketch33" plane through (19.6, 13.8, 2.2) normal (0, 0, -1) x (-1, 0, 0)
  line L0 (0, -10.2) -> (0, 0) construction
  line L1 (0, 0) -> (-123.7858, 0) construction
  line L2 (0, 0) -> (-0.7071, -0.7071) construction
  circle A0 centre (-0.7071, -0.7071) radius 1
  dimension "d329" = 1
  constraint coincident L0.end L1.start
  constraint coincident L0.end A0
  measures "d329" distance of L0.end L2.end
sweep "Sweep31" cut kept parallel profiles "Sketch33" along 1 edges at (19.6, 13.8, 1.2) section 1
ref_plane "WorkPlane32" through (19.6, 3.6, 2.2) normal (0, 0, -1) x (-1, 0, 0)
sketch "Sketch34" plane through (19.6, 3.6, 2.2) normal (0, 0, -1) x (-1, 0, 0)
  line L0 (-123.7858, 0) -> (0, 0) construction
  line L1 (0, 0) -> (0, 8.7858) construction
  line L2 (0, 0) -> (-0.7071, 0.7071) construction
  circle A0 centre (-0.7071, 0.7071) radius 1
  dimension "d337" = 1
  constraint coincident L0.end L1.start
  constraint coincident L0.end A0
  measures "d337" distance of L0.end L2.end
sweep "Sweep32" cut kept parallel profiles "Sketch34" along 1 edges at (19.6, 3.6, 1.2) section 1
extrude "Extrude3" cut sketch "Sketch2" against normal blind 2.2 contours L2 L3 L103 L104 L105
extrude "Extrude4" add sketch "Sketch2" along normal blind 1.6 contours L45 L46 L47 L48 L49 L50 L51 L52 | L53 L54 L55 | L56 L58 L70 L75 | L56 L58 L66 L71 | L56 L58 L63 L67 | A0 | A1 | A2 | L78 L80 L81 L89 | L78 L86 L87 L89 | L78 L80 L87 L89 | L78 L80 L87 L92 | L80 L82 L87 L89 | L78 L90 L91 L92 | L78 L80 L90 L92 | L82 L83 L84 L89 | L82 L84 L87 L89 | L78 L80 L90 L96 | L80 L82 L90 L92 | L82 L84 L87 L92 | L84 L87 L88 L89 | L78 L94 L95 L96 | L78 L80 L94 L96 | L82 L84 L90 L92 | L78 L79 L80 L94 | L80 L82 L94 L96 | L82 L84 L90 L96 | L84 L90 L92 L93 | L82 L84 L94 L96 | L82 L84 L85 L94 | L84 L94 L96 L97 | L98 L99 L100 A3
extrude "Extrude5" add sketch "Sketch2" along normal blind 3.2 contours L56 L58 L59 L74 L75 L76 L77 | L56 L58 L70 L71 L72 L73 | L56 L58 L66 L67 L68 L69 | L56 L57 L58 L62 L63 L64 L65
ref_plane "WorkPlane33" through (9.8, 0, 0) normal (1, 0, 0) x (0, 1, 0)
sketch "Sketch35" plane through (9.8, 0, 0) normal (1, 0, 0) x (0, 1, 0)
  line L0 (69.7, 2.2) -> (72.7, 2.2)
  line L1 (72.7, 2.2) -> (72.7, 5.4)
  line L2 (69.7, 2.2) -> (66.7, 2.2)
  line L3 (66.7, 2.2) -> (66.7, 3.8)
  line L4 (72.7, 5.4) -> (66.7, 3.8)
  line L5 (57.5, 2.2) -> (60.5, 2.2)
  line L6 (60.5, 2.2) -> (60.5, 3.8)
  line L7 (57.5, 2.2) -> (54.5, 2.2)
  line L8 (54.5, 2.2) -> (54.5, 3.8)
  line L9 (57.5, 2.2) -> (57.5, 3.8) construction
  arc A0 (60.5, 3.8) -> (54.5, 3.8) centre (57.5, 3.8) ccw
  point P0 (69.7, 2.2)
  point P1 (57.5, 2.2)
  dimension "d351" = 3
  dimension "d352" = 3.2
  dimension "d353" = 3
  dimension "d354" = 1.6
  dimension "d355" = 3
  dimension "d356" = 1.6
  dimension "d357" = 3
  dimension "d358" = 1.6
  dimension "d359" = 1.6
  constraint coincident P0 L0.start
  constraint perpendicular L0 L1
  constraint parallel L0 L2
  constraint perpendicular L2 L3
  constraint coincident P1 L5.start
  constraint perpendicular L3 L5
  constraint perpendicular L5 L6
  constraint parallel L5 L7
  constraint perpendicular L7 L8
  constraint perpendicular L7 L9
  constraint coincident L9.end A0.centre
  measures "d351" distance of P0 L0.end
  measures "d352" distance of L0.end L1.end
  measures "d353" distance of P0 L2.end
  measures "d354" distance of L2.end L3.end
  measures "d355" distance of P1 L5.end
  measures "d356" distance of L5.end L6.end
  measures "d357" distance of P1 L7.end
  measures "d358" distance of L7.end L8.end
  measures "d359" distance of P1 L9.end
extrude "Extrude6" add sketch "Sketch35" along normal mid plane 6
equation "length_Ref = 170 mm" comment "Side lengths of base of model"
equation "baseHeight_Ref = 0.4 mm" comment "Height of the base of the model"
equation "sidewalkHeight_Ref = 3.2 mm" comment "Height of sidewalk/walking surface"
equation "sidewalkWidth_Ref = length_Ref / 3" comment "Width of the sidewalk/walking surface"
equation "orientorSize_Ref = 6 mm" comment "Side length of orientation indicator square"
equation "oritentorHeight_Ref = 2.4 mm" comment "Height of the orientation indicator"
equation "braileHeight_Ref = 0.6 mm" comment "Standard height of Braille characters"
equation "filletRadius_Ref = 0.6 mm" comment "Radius of fillets to soften edges"
equation "lineWidth_Ref = 3 mm" comment "Width of crosswalk lines"
equation "lineHeight_Ref = braileHeight_Ref / 2" comment "Height of crosswalk lines"
equation "tabWidth_Ref = length_Ref / 10" comment "Width of tabs to secure adjacent maps together"
equation "tabLength_Ref = length_Ref / 14" comment "Length of tab to secure adjacent maps together"
equation "tabHeight_Ref = sidewalkHeight_Ref / 4" comment "Height of tabs to secure adjacent maps together"
equation "clearance_Ref = 0.2 mm" comment "Clearance around parts that will fit together"
equation "featureHeight_Ref = 1.6 mm" comment "Height of features such as bus stops"
equation "pegSize_Ref = 6 mm" comment "Side length of pegs/holes to connect features to map base"
equation "pegDepth_Ref = sidewalkHeight_Ref / 4" comment "Depth of pegs/holes to connect features to map base"
equation "dogbone_Ref = 2 mm" comment "\"Cutter\" diameter for creating dogbone corners."
equation "labelHeight = 10 mm + clearance_Ref" comment "Height of the braille labels with clearance"
equation "labelSpacing = 2 mm" comment "Spacing between labels"
equation "d21 = 139 mm + 8.25 mm"
equation "d26 = 25 mm + clearance_Ref + 6.25 mm"
equation "d27 = labelHeight"
equation "d28 = labelSpacing"
equation "d29 = 31.25 mm + 6.25 mm + clearance_Ref"
equation "d30 = labelSpacing"
equation "d31 = labelHeight"
equation "d32 = 43.75 mm + 6.25 mm + clearance_Ref"
equation "d33 = labelHeight"
equation "d34 = labelSpacing"
equation "d35 = 50 mm + 6.25 mm + clearance_Ref"
equation "d36 = labelHeight"
equation "d37 = labelSpacing"
equation "d38 = 56.25 mm + 6.25 mm + clearance_Ref"
equation "d39 = labelHeight"
equation "d40 = labelSpacing"
equation "d41 = 62.5 mm + 6.25 mm + clearance_Ref"
equation "d42 = labelHeight"
equation "d43 = labelSpacing"
equation "d44 = 81.25 mm + 6.25 mm + clearance_Ref"
equation "d45 = labelHeight"
equation "d46 = labelSpacing"
equation "d47 = 118.75 mm + 6.25 mm + clearance_Ref"
equation "d48 = labelHeight"
equation "d49 = labelSpacing"
equation "d50 = ( 19.6 / 2 ) * 1 mm"
equation "d51 = pegSize_Ref / 2"
equation "d52 = pegSize_Ref / 2"
equation "d53 = 2 * pegSize_Ref"
equation "d54 = pegSize_Ref"
equation "d55 = pegSize_Ref / 4"
equation "d56 = pegSize_Ref"
equation "d59 = -pegSize_Ref * 2 + pegSize_Ref / 4"
equation "d61 = pegSize_Ref / 4"
equation "d64 = pegSize_Ref / 2"
equation "d66 = pegSize_Ref * 2"
equation "d67 = pegSize_Ref / 4"
equation "d68 = pegSize_Ref"
equation "d69 = pegSize_Ref / 2 - pegSize_Ref / 12"
equation "d70 = pegSize_Ref / 4"
equation "d71 = pegSize_Ref"
equation "d72 = pegSize_Ref / 12"
equation "d73 = pegSize_Ref / 6"
equation "d78 = pegSize_Ref"
equation "d83 = pegSize_Ref / 3"
equation "d84 = pegSize_Ref / 6"
equation "d85 = pegSize_Ref"
equation "d89 = dogbone_Ref / 2"
equation "d97 = dogbone_Ref / 2"
equation "d105 = dogbone_Ref / 2"
equation "d113 = dogbone_Ref / 2"
equation "d121 = dogbone_Ref / 2"
equation "d129 = dogbone_Ref / 2"
equation "d137 = dogbone_Ref / 2"
equation "d145 = dogbone_Ref / 2"
equation "d153 = dogbone_Ref / 2"
equation "d161 = dogbone_Ref / 2"
equation "d169 = dogbone_Ref / 2"
equation "d177 = dogbone_Ref / 2"
equation "d185 = dogbone_Ref / 2"
equation "d193 = dogbone_Ref / 2"
equation "d201 = dogbone_Ref / 2"
equation "d209 = dogbone_Ref / 2"
equation "d217 = dogbone_Ref / 2"
equation "d225 = dogbone_Ref / 2"
equation "d233 = dogbone_Ref / 2"
equation "d241 = dogbone_Ref / 2"
equation "d249 = dogbone_Ref / 2"
equation "d257 = dogbone_Ref / 2"
equation "d265 = dogbone_Ref / 2"
equation "d273 = dogbone_Ref / 2"
equation "d281 = dogbone_Ref / 2"
equation "d289 = dogbone_Ref / 2"
equation "d297 = dogbone_Ref / 2"
equation "d305 = dogbone_Ref / 2"
equation "d313 = dogbone_Ref / 2"
equation "d321 = dogbone_Ref / 2"
equation "d329 = dogbone_Ref / 2"
equation "d337 = dogbone_Ref / 2"
equation "d346 = featureHeight_Ref"
equation "d348 = 2 * featureHeight_Ref"
equation "d350 = ( 19.6 / 2 ) * 1 mm"
equation "d351 = pegSize_Ref / 2"
equation "d352 = featureHeight_Ref * 2"
equation "d353 = pegSize_Ref / 2"
equation "d354 = featureHeight_Ref"
equation "d355 = pegSize_Ref / 2"
equation "d356 = featureHeight_Ref"
equation "d357 = pegSize_Ref / 2"
equation "d358 = featureHeight_Ref"
equation "d359 = featureHeight_Ref"
equation "d360 = pegSize_Ref / 2"
